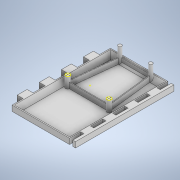
# Autodesk Inventor part: rfid_top
Saved by Autodesk Inventor 2020 (Build 240168000, 168)
## iProperties
Created: 2019-06-30
Part Number: rfid_top
Material: Generic
Document SubType Name: Modeling
Designer: jjsch
Density: 1 g/cm^3
Appearance: Default
Mass: 12.4406 g
Surface Area: 151.295 cm^2
Volume: 12.4406 cm^3
Author: jjsch
Autodesk Inventor part; units mm, degrees
ref_plane "YZ Plane" through (0, 0, 0) normal (1, 0, 0) x (0, 1, 0)
ref_plane "XZ Plane" through (0, 0, 0) normal (0, 1, 0) x (-1, 0, 0)
ref_plane "XY Plane" through (0, 0, 0) normal (0, 0, 1) x (1, 0, 0)
sketch "Sketch1" plane through (0, 0, 0) normal (0, 1, 0) x (-1, 0, 0)
  line L0 (-31.9185, 45) -> (31.9185, 45)
  line L1 (31.9185, 45) -> (31.9185, -45)
  line L2 (31.9185, -45) -> (-31.9185, -45)
  line L3 (-31.9185, -45) -> (-31.9185, 45)
  line L4 (-31.9185, 45) -> (31.9185, -45) construction
  line L5 (31.9185, 45) -> (-31.9185, -45) construction
  point P0 (0, 0)
  dimension "d0" = 63.837
  dimension "d1" = 90
  constraints: 12 end point, 2 midpoint, 2 parallel, 1 horizontal, 1 perpendicular
  measures "d0" distance of L1.end L2.end
  measures "d1" distance of L0.end L1.end
extrude "Extrusion1" add sketch "Sketch1" along normal blind 5
sketch "Sketch2" plane through (0, 5, 0) normal (0, 1, 0) x (1, 0, 0)
  line L0 (31.9185, -45) -> (31.9185, 45) projected
  line L1 (31.9185, -45) -> (26.4995, -45)
  line L2 (26.4995, -45) -> (26.4995, -35)
  line L3 (26.4995, -35) -> (31.9185, -35)
  line L4 (31.9185, -35) -> (31.9185, -45)
  line L5 (-31.9185, 45) -> (-31.9185, -45) projected
  line L6 (-31.9185, -45) -> (-26.4995, -45)
  line L7 (-26.4995, -45) -> (-26.4995, -35)
  line L8 (-26.4995, -35) -> (-31.9185, -35)
  line L9 (-31.9185, -35) -> (-31.9185, -45)
  line L10 (31.9185, -25) -> (26.4995, -25)
  line L11 (26.4995, -25) -> (26.4995, -15)
  line L12 (26.4995, -15) -> (31.9185, -15)
  line L13 (31.9185, -15) -> (31.9185, -25)
  line L14 (-31.9185, -25) -> (-26.4995, -25)
  line L15 (-26.4995, -25) -> (-26.4995, -15)
  line L16 (-26.4995, -15) -> (-31.9185, -15)
  line L17 (-31.9185, -15) -> (-31.9185, -25)
  line L18 (31.9185, -5) -> (26.4995, -5)
  line L19 (26.4995, -5) -> (26.4995, 5)
  line L20 (26.4995, 5) -> (31.9185, 5)
  line L21 (31.9185, 5) -> (31.9185, -5)
  line L22 (-31.9185, -5) -> (-26.4995, -5)
  line L23 (-26.4995, -5) -> (-26.4995, 5)
  line L24 (-26.4995, 5) -> (-31.9185, 5)
  line L25 (-31.9185, 5) -> (-31.9185, -5)
  line L26 (31.9185, 15) -> (26.4995, 15)
  line L27 (26.4995, 15) -> (26.4995, 25)
  line L28 (26.4995, 25) -> (31.9185, 25)
  line L29 (31.9185, 25) -> (31.9185, 15)
  line L30 (-31.9185, 15) -> (-26.4995, 15)
  line L31 (-26.4995, 15) -> (-26.4995, 25)
  line L32 (-26.4995, 25) -> (-31.9185, 25)
  line L33 (-31.9185, 25) -> (-31.9185, 15)
  line L34 (31.9185, 35) -> (26.4995, 35)
  line L35 (26.4995, 35) -> (26.4995, 45)
  line L36 (26.4995, 45) -> (31.9185, 45)
  line L37 (31.9185, 45) -> (31.9185, 35)
  line L38 (-31.9185, 35) -> (-26.4995, 35)
  line L39 (-26.4995, 35) -> (-26.4995, 45)
  line L40 (-26.4995, 45) -> (-31.9185, 45)
  line L41 (-31.9185, 45) -> (-31.9185, 35)
  point P0 (0, 0)
  dimension "d4" = 5.419
  dimension "d5" = 10
  dimension "d6" = 5.419
  dimension "d7" = 10
  dimension "d10" = 20
  constraints: 80 end point, 4 parallel, 2 horizontal, 2 perpendicular, 1 vertical, 64 other
  measures "d4" distance of L2.end L3.end
  measures "d5" distance of L1.end L2.end
  measures "d6" distance of L8.end L7.end
  measures "d7" distance of L7.end L6.end
  measures "d10" distance of L2.end L11.end
extrude "Extrusion2" cut sketch "Sketch2" against normal blind 5
sketch "Sketch3" plane through (0, 5, 0) normal (0, 1, 0) x (1, 0, 0)
  line L0 (28.4995, -45) -> (31.9185, -45)
  line L1 (31.9185, -45) -> (31.9185, 45)
  line L2 (31.9185, 45) -> (28.4995, 45)
  line L3 (28.4995, 45) -> (28.4995, -45)
  line L4 (-26.4995, -45) -> (26.4995, -45) projected
  line L5 (26.4995, -45) -> (26.4995, -35) projected
  point P0 (0, 0)
  dimension "d17" = 90
  dimension "d18" = 3.419
  dimension "d19" = 0
  dimension "d20" = 2
  constraints: 8 end point, 2 parallel, 1 horizontal, 1 perpendicular
  measures "d17" distance of L1.end L0.end
  measures "d18" distance of L0.start L0.end
  measures "d19" distance between parallel lines of L4 L0
  measures "d20" distance between parallel lines of L5 L3
extrude "Extrusion3" add sketch "Sketch3" against normal blind 5
sketch "Sketch4" plane through (0, 5, 0) normal (0, 1, 0) x (1, 0, 0)
  line L0 (31.9185, -45) -> (31.9185, 45) projected
  line L1 (31.9185, 45) -> (28.4995, 45) projected
  line L2 (28.4995, 45) -> (28.4995, 35) projected
  line L3 (28.4995, 35) -> (26.4995, 35) projected
  line L4 (26.4995, 35) -> (26.4995, 45) projected
  line L5 (26.4995, 45) -> (-26.4995, 45) projected
  line L6 (-26.4995, 45) -> (-26.4995, 35) projected
  line L7 (-26.4995, 35) -> (-31.9185, 35) projected
  line L8 (-31.9185, 35) -> (-31.9185, 25) projected
  line L9 (-31.9185, 25) -> (-26.4995, 25) projected
  line L10 (-26.4995, 25) -> (-26.4995, 15) projected
  line L11 (-26.4995, 15) -> (-31.9185, 15) projected
  line L12 (-31.9185, 15) -> (-31.9185, 5) projected
  line L13 (-31.9185, 5) -> (-26.4995, 5) projected
  line L14 (-26.4995, 5) -> (-26.4995, -5) projected
  line L15 (-26.4995, -5) -> (-31.9185, -5) projected
  line L16 (-31.9185, -5) -> (-31.9185, -15) projected
  line L17 (-31.9185, -15) -> (-26.4995, -15) projected
  line L18 (-26.4995, -15) -> (-26.4995, -25) projected
  line L19 (-26.4995, -25) -> (-31.9185, -25) projected
  line L20 (-31.9185, -25) -> (-31.9185, -35) projected
  line L21 (-31.9185, -35) -> (-26.4995, -35) projected
  line L22 (-26.4995, -35) -> (-26.4995, -45) projected
  line L23 (-26.4995, -45) -> (26.4995, -45) projected
  line L24 (26.4995, -45) -> (26.4995, -35) projected
  line L25 (26.4995, -35) -> (28.4995, -35) projected
  line L26 (28.4995, -35) -> (28.4995, -45) projected
  line L27 (28.4995, -45) -> (31.9185, -45) projected
  line L28 (28.4995, 25) -> (28.4995, 15) projected
  line L29 (28.4995, 15) -> (26.4995, 15) projected
  line L30 (26.4995, 15) -> (26.4995, 25) projected
  line L31 (26.4995, 25) -> (28.4995, 25) projected
  line L32 (28.4995, 5) -> (28.4995, -5) projected
  line L33 (28.4995, -5) -> (26.4995, -5) projected
  line L34 (26.4995, -5) -> (26.4995, 5) projected
  line L35 (26.4995, 5) -> (28.4995, 5) projected
  line L36 (28.4995, -15) -> (28.4995, -25) projected
  line L37 (28.4995, -25) -> (26.4995, -25) projected
  line L38 (26.4995, -25) -> (26.4995, -15) projected
  line L39 (26.4995, -15) -> (28.4995, -15) projected
  line L40 (-20.9995, 39.5) -> (20.9995, 39.5)
  line L41 (20.9995, 39.5) -> (20.9995, 29.5)
  line L42 (20.9995, 29.5) -> (26.4185, 29.5)
  line L43 (26.4185, 29.5) -> (26.4185, -29.5)
  line L44 (26.4185, -29.5) -> (20.9995, -29.5)
  line L45 (20.9995, -29.5) -> (20.9995, -39.5)
  line L46 (20.9995, -39.5) -> (-20.9995, -39.5)
  line L47 (-20.9995, -39.5) -> (-20.9995, -30.5)
  line L48 (-20.9995, -30.5) -> (-20.9995, -10.5)
  line L49 (-20.9995, -10.5) -> (-20.9995, 9.5)
  line L50 (-20.9995, 9.5) -> (-20.9995, 29.5)
  line L51 (-20.9995, 29.5) -> (-20.9995, 39.5)
  line L52 (20.9995, 29.5) -> (20.9995, -29.5)
  point P0 (0, 0)
  dimension "d23" = 5.5
  constraints: 26 end point, 1 collinear, 11 other
  measures "d23" distance between parallel lines of L5 L40
extrude "Extrusion4" cut sketch "Sketch4" against normal blind 4 contours L40 L41 L52 L45 L46 L47 L48 L49 L50 L51
chamfer "Chamfer1" distance 4 angle 45 4 edges at (-20.9995, 5, 0) (0, 5, -39.5) (20.9995, 5, 0) (0, 5, 39.5)
sketch "Sketch5" plane through (0, 0, 0) normal (0, -1, 0) x (1, 0, 0)
  circle A0 centre (-13.95, -41) radius 1.6
  circle A1 centre (13.95, -41) radius 1.6
  circle A2 centre (-18.65, 1.5) radius 1.9
  circle A3 centre (18.65, 1.5) radius 1.9
  line L0 (-26.4995, 45) -> (26.4995, 45) projected
  line L1 (26.4995, -45) -> (-26.4995, -45) projected
  point P0 (0, 0)
  dimension "d29" = 3.2
  dimension "d30" = 3.2
  dimension "d31" = 27.9
  dimension "d32" = 13.95
  dimension "d33" = 3.8
  dimension "d34" = 3.8
  dimension "d37" = 42.5
  dimension "d39" = 4.7
  dimension "d40" = 4.7
  dimension "d41" = 43.5
  dimension "d42" = 4
  constraints: 4 centre point, 2 horizontal alignment
  measures "d29" diameter of A0
  measures "d30" diameter of A1
  measures "d31" distance of A1.centre A0.centre
  measures "d32" horizontal distance of point (0, 0) A1.centre
  measures "d33" diameter of A2
  measures "d34" diameter of A3
  measures "d37" vertical distance of A0.centre A2.centre
  measures "d39" horizontal distance of A2.centre A0.centre
  measures "d40" horizontal distance of A3.centre A1.centre
  measures "d41" distance from line of L0 A2.centre
  measures "d42" distance from line of L1 A0.centre
extrude "Extrusion5" add sketch "Sketch5" against normal blind 15
sketch "Sketch6" plane through (0, 1, 0) normal (0, 1, 0) x (1, 0, 0)
  circle A0 centre (18.65, -1.5) radius 1.9 projected
  circle A1 centre (-18.65, -1.5) radius 1.9 projected
  circle A2 centre (-13.95, 41) radius 1.6 projected
  circle A3 centre (13.95, 41) radius 1.6 projected
  line L0 (18.65, -1.5) -> (-18.65, -1.5)
  arc A4 (14.5068, 39.5) -> (13.3932, 39.5) centre (13.95, 41) ccw projected
  line L1 (18.65, -1.5) -> (13.95, 41)
  line L2 (-13.95, 41) -> (-18.65, -1.5)
  arc A5 (-13.3932, 39.5) -> (-14.5068, 39.5) centre (-13.95, 41) ccw projected
  line L3 (-13.6021, 40.9615) -> (-18.3021, -1.5385)
  line L4 (-18.3021, -1.5385) -> (-18.9979, -1.4615)
  line L5 (-18.9979, -1.4615) -> (-14.2979, 41.0385)
  line L6 (-14.2979, 41.0385) -> (-13.6021, 40.9615)
  line L7 (-13.6021, 40.9615) -> (-18.9979, -1.4615) construction
  line L8 (-18.3021, -1.5385) -> (-14.2979, 41.0385) construction
  line L9 (-17.05, -1.15) -> (17.05, -1.15)
  line L10 (17.05, -1.15) -> (17.05, -1.85)
  line L11 (17.05, -1.85) -> (-17.05, -1.85)
  line L12 (-17.05, -1.85) -> (-17.05, -1.15)
  line L13 (-17.05, -1.15) -> (17.05, -1.85) construction
  line L14 (17.05, -1.15) -> (-17.05, -1.85) construction
  line L15 (19.0356, -1.8031) -> (14.2601, 41.38)
  line L16 (14.2601, 41.38) -> (13.5644, 41.3031)
  line L17 (13.5644, 41.3031) -> (18.3399, -1.88)
  line L18 (18.3399, -1.88) -> (19.0356, -1.8031)
  line L19 (19.0356, -1.8031) -> (13.5644, 41.3031) construction
  line L20 (14.2601, 41.38) -> (18.3399, -1.88) construction
  line L21 (14.2987, 41.73) -> (-14.2987, 41.73)
  line L22 (-14.2987, 41.73) -> (-14.2987, 41.03)
  line L23 (-14.2987, 41.03) -> (14.2987, 41.03)
  line L24 (14.2987, 41.03) -> (14.2987, 41.73)
  line L25 (14.2987, 41.73) -> (-14.2987, 41.03) construction
  line L26 (-14.2987, 41.73) -> (14.2987, 41.03) construction
  point P0 (0, 0)
  point P1 (0, 41)
  point P2 (-16.3, 19.75)
  point P3 (0, -1.5)
  point P4 (16.3, 19.75)
  point P5 (-17.05, -1.5)
  point P6 (16.7366, -1.85)
  point P7 (17.0113, -1.85)
  point P8 (17.05, -1.8457)
  point P9 (16.6592, -1.15)
  point P10 (-16.6592, -1.15)
  point P11 (0, 41.38)
  point P12 (14.2987, 41.0313)
  point P13 (-14.2987, 41.0313)
  point P14 (-14.2214, 41.03)
  point P15 (13.5945, 41.03)
  dimension "d46" = 0.7
  dimension "d47" = 0.7
  dimension "d48" = 0.7
  dimension "d53" = 0.7
  dimension "d54" = 0.7
  constraints: 54 end point, 11 midpoint, 10 parallel, 4 perpendicular, 3 horizontal, 1 point on line
  measures "d46" distance of L3.end L4.end
  measures "d47" distance of L9.end L10.end
  measures "d48" distance of L16.end L15.end
  measures "d53" distance between parallel lines of L11 L9
  measures "d54" distance of L22.end L21.end
extrude "Extrusion6" add sketch "Sketch6" along normal blind 5 contours L15 L18 L17 L0 L1 A0 | A0 L1 A3 L15 | L11 A1 L0 A0 | A0 L0 L10 L11 | L1 L0 L17 A0 | A0 L17 A3 L1 | A3 L17 L23 L15 | L0 A1 L9 A0 | A0 L9 L10 L0 | L11 L12 L0 A1 | L23 L17 L16 L15 | L15 L16 L17 L23 A3 L21 L24 | L0 L12 L9 A1 | L5 A2 L2 A1 | A1 L2 L4 L5 | L2 A2 L3 A1 | A1 L3 L0 L2 | L5 L23 L6 L2 A2 | A3 L23 A2 L21 | L3 L4 L0 | L2 L6 L3 A2 | L5 L6 L23 | A2 L23 L6 L22 L21
sketch "Sketch7" plane through (18.65, 15, 1.5) normal (0, 1, 0) x (1, 0, 0)
  circle A0 centre (-37.3, 0) radius 1.9 projected
  circle A1 centre (0, 0) radius 1.9 projected
  point P0 (-18.65, 1.5)
extrude "Extrusion7" cut sketch "Sketch7" against normal blind 4
sketch "Sketch8" plane through (-18.65, 11, 1.5) normal (0, 1, 0) x (1, 0, 0)
  circle A0 centre (37.3, 0) radius 1.9 projected
  circle A1 centre (0, 0) radius 1.9 projected
  point P0 (18.65, 1.5)
  constraints: 2 coincident
sketch "Sketch9" plane through (0, 5, 0) normal (0, 1, 0) x (1, 0, 0)
  line L0 (28.4995, -15) -> (28.4995, -25) projected
  line L1 (28.4995, -25) -> (26.4995, -25) projected
  line L2 (26.4995, -25) -> (26.4995, -15) projected
  line L3 (26.4995, -15) -> (28.4995, -15) projected
  line L4 (28.4995, 5) -> (28.4995, -5) projected
  line L5 (28.4995, -5) -> (26.4995, -5) projected
  line L6 (26.4995, -5) -> (26.4995, 5) projected
  line L7 (26.4995, 5) -> (28.4995, 5) projected
  line L8 (28.4995, 25) -> (28.4995, 15) projected
  line L9 (28.4995, 15) -> (26.4995, 15) projected
  line L10 (26.4995, 15) -> (26.4995, 25) projected
  line L11 (26.4995, 25) -> (28.4995, 25) projected
  line L12 (31.9185, -45) -> (31.9185, 45) projected
  line L13 (31.9185, 45) -> (28.4995, 45) projected
  line L14 (28.4995, 45) -> (28.4995, 35) projected
  line L15 (28.4995, 35) -> (26.4995, 35) projected
  line L16 (26.4995, 35) -> (26.4995, 45) projected
  line L17 (26.4995, 45) -> (-26.4995, 45) projected
  line L18 (-26.4995, 45) -> (-26.4995, 35) projected
  line L19 (-26.4995, 35) -> (-31.9185, 35) projected
  line L20 (-31.9185, 35) -> (-31.9185, 25) projected
  line L21 (-31.9185, 25) -> (-26.4995, 25) projected
  line L22 (-26.4995, 25) -> (-26.4995, 15) projected
  line L23 (-26.4995, 15) -> (-31.9185, 15) projected
  line L24 (-31.9185, 15) -> (-31.9185, 5) projected
  line L25 (-31.9185, 5) -> (-26.4995, 5) projected
  line L26 (-26.4995, 5) -> (-26.4995, -5) projected
  line L27 (-26.4995, -5) -> (-31.9185, -5) projected
  line L28 (-31.9185, -5) -> (-31.9185, -15) projected
  line L29 (-31.9185, -15) -> (-26.4995, -15) projected
  line L30 (-26.4995, -15) -> (-26.4995, -25) projected
  line L31 (-26.4995, -25) -> (-31.9185, -25) projected
  line L32 (-31.9185, -25) -> (-31.9185, -35) projected
  line L33 (-31.9185, -35) -> (-26.4995, -35) projected
  line L34 (-26.4995, -35) -> (-26.4995, -45) projected
  line L35 (-26.4995, -45) -> (26.4995, -45) projected
  line L36 (26.4995, -45) -> (26.4995, -35) projected
  line L37 (26.4995, -35) -> (28.4995, -35) projected
  line L38 (28.4995, -35) -> (28.4995, -45) projected
  line L39 (28.4995, -45) -> (31.9185, -45) projected
  line L40 (24.9995, 43.5) -> (-24.9995, 43.5) projected
  line L41 (24.9995, -43.5) -> (24.9995, 43.5) projected
  line L42 (-24.9995, -43.5) -> (24.9995, -43.5) projected
  line L43 (-24.9995, 43.5) -> (-24.9995, -43.5) projected
  line L44 (31.4185, 44.5) -> (31.4185, -44.5)
  line L45 (31.4185, -44.5) -> (28.9995, -44.5)
  line L46 (28.9995, -44.5) -> (28.9995, -34.5)
  line L47 (28.9995, -34.5) -> (25.9995, -34.5)
  line L48 (25.9995, -34.5) -> (25.9995, -44.5)
  line L49 (25.9995, -44.5) -> (-25.9995, -44.5)
  line L50 (-25.9995, -44.5) -> (-25.9995, -34.5)
  line L51 (-25.9995, -34.5) -> (-31.4185, -34.5)
  line L52 (-31.4185, -34.5) -> (-31.4185, -25.5)
  line L53 (-31.4185, -25.5) -> (-25.9995, -25.5)
  line L54 (-25.9995, -25.5) -> (-25.9995, -14.5)
  line L55 (-25.9995, -14.5) -> (-31.4185, -14.5)
  line L56 (-31.4185, -14.5) -> (-31.4185, -5.5)
  line L57 (-31.4185, -5.5) -> (-25.9995, -5.5)
  line L58 (-25.9995, -5.5) -> (-25.9995, 5.5)
  line L59 (-25.9995, 5.5) -> (-31.4185, 5.5)
  line L60 (-31.4185, 5.5) -> (-31.4185, 14.5)
  line L61 (-31.4185, 14.5) -> (-25.9995, 14.5)
  line L62 (-25.9995, 14.5) -> (-25.9995, 25.5)
  line L63 (-25.9995, 25.5) -> (-31.4185, 25.5)
  line L64 (-31.4185, 25.5) -> (-31.4185, 34.5)
  line L65 (-31.4185, 34.5) -> (-25.9995, 34.5)
  line L66 (-25.9995, 34.5) -> (-25.9995, 44.5)
  line L67 (-25.9995, 44.5) -> (25.9995, 44.5)
  line L68 (25.9995, 44.5) -> (25.9995, 34.5)
  line L69 (25.9995, 34.5) -> (28.9995, 34.5)
  line L70 (28.9995, 34.5) -> (28.9995, 44.5)
  line L71 (28.9995, 44.5) -> (31.4185, 44.5)
  line L72 (28.9995, -25.5) -> (28.9995, -14.5)
  line L73 (28.9995, -14.5) -> (25.9995, -14.5)
  line L74 (25.9995, -14.5) -> (25.9995, -25.5)
  line L75 (25.9995, -25.5) -> (28.9995, -25.5)
  line L76 (28.9995, -5.5) -> (28.9995, 5.5)
  line L77 (28.9995, 5.5) -> (25.9995, 5.5)
  line L78 (25.9995, 5.5) -> (25.9995, -5.5)
  line L79 (25.9995, -5.5) -> (28.9995, -5.5)
  line L80 (25.9995, 25.5) -> (25.9995, 14.5)
  line L81 (25.9995, 14.5) -> (28.9995, 14.5)
  line L82 (28.9995, 14.5) -> (28.9995, 25.5)
  line L83 (28.9995, 25.5) -> (25.9995, 25.5)
  line L84 (28.4995, -15) -> (28.4995, -25) projected
  line L85 (28.4995, -25) -> (26.4995, -25) projected
  line L86 (26.4995, -25) -> (26.4995, -15) projected
  line L87 (26.4995, -15) -> (28.4995, -15) projected
  line L88 (28.4995, 5) -> (28.4995, -5) projected
  line L89 (28.4995, -5) -> (26.4995, -5) projected
  line L90 (26.4995, -5) -> (26.4995, 5) projected
  line L91 (26.4995, 5) -> (28.4995, 5) projected
  line L92 (28.4995, 25) -> (28.4995, 15) projected
  line L93 (28.4995, 15) -> (26.4995, 15) projected
  line L94 (26.4995, 15) -> (26.4995, 25) projected
  line L95 (26.4995, 25) -> (28.4995, 25) projected
  line L96 (31.9185, -45) -> (31.9185, 45) projected
  line L97 (31.9185, 45) -> (28.4995, 45) projected
  line L98 (28.4995, 45) -> (28.4995, 35) projected
  line L99 (28.4995, 35) -> (26.4995, 35) projected
  line L100 (26.4995, 35) -> (26.4995, 45) projected
  line L101 (26.4995, 45) -> (-26.4995, 45) projected
  line L102 (-26.4995, 45) -> (-26.4995, 35) projected
  line L103 (-26.4995, 35) -> (-31.9185, 35) projected
  line L104 (-31.9185, 35) -> (-31.9185, 25) projected
  line L105 (-31.9185, 25) -> (-26.4995, 25) projected
  line L106 (-26.4995, 25) -> (-26.4995, 15) projected
  line L107 (-26.4995, 15) -> (-31.9185, 15) projected
  line L108 (-31.9185, 15) -> (-31.9185, 5) projected
  line L109 (-31.9185, 5) -> (-26.4995, 5) projected
  line L110 (-26.4995, 5) -> (-26.4995, -5) projected
  line L111 (-26.4995, -5) -> (-31.9185, -5) projected
  line L112 (-31.9185, -5) -> (-31.9185, -15) projected
  line L113 (-31.9185, -15) -> (-26.4995, -15) projected
  line L114 (-26.4995, -15) -> (-26.4995, -25) projected
  line L115 (-26.4995, -25) -> (-31.9185, -25) projected
  line L116 (-31.9185, -25) -> (-31.9185, -35) projected
  line L117 (-31.9185, -35) -> (-26.4995, -35) projected
  line L118 (-26.4995, -35) -> (-26.4995, -45) projected
  line L119 (-26.4995, -45) -> (26.4995, -45) projected
  line L120 (26.4995, -45) -> (26.4995, -35) projected
  line L121 (26.4995, -35) -> (28.4995, -35) projected
  line L122 (28.4995, -35) -> (28.4995, -45) projected
  line L123 (28.4995, -45) -> (31.9185, -45) projected
  line L124 (24.9995, 43.5) -> (-24.9995, 43.5) projected
  line L125 (24.9995, -43.5) -> (24.9995, 43.5) projected
  line L126 (-24.9995, -43.5) -> (24.9995, -43.5) projected
  line L127 (-24.9995, 43.5) -> (-24.9995, -43.5) projected
  point P0 (0, 0)
  dimension "d55" = 0.5
  dimension "d56" = 0.5
  dimension "d57" = 0.5
  dimension "d58" = 0.5
  constraints: 80 end point, 36 other
  measures "d55" distance between parallel lines of L12 L44
  measures "d56" distance between parallel lines of L0 L72
  measures "d57" distance between parallel lines of L4 L76
  measures "d58" distance between parallel lines of L10 L80
extrude "Tolerances Extrusion" cut sketch "Sketch9" against normal blind 5 contours L0 L1 L2 L3 | L4 L5 L6 L7 | L8 L9 L10 L11 | L39 L38 L37 L36 L35 L34 L33 L32 L31 L30 L29 L28 L27 L26 L25 L24 L23 L22 L21 L20 L19 L18 L17 L16 L15 L14 L13 L12 | L75 L74 L73 L72 | L79 L78 L77 L76 | L83 L82 L81 L80
body "Solid1"
